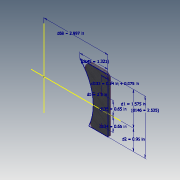
# Autodesk Inventor part: J005357
Saved by Autodesk Inventor 2015 SP1 (Build 190203100, 203)
## iProperties
Created: 2015-07-20
Material: STEEL, LOW CARBON (1008/1018/1020)
Vendor: HHMI: JRC - ID&F
Document SubType Name: Modeling
Designer: ARNOLDJ
Density: 7.85 g/cm^3
Appearance: Metal-Steel (Machined_00)
Mass: 17.3845 g
Surface Area: 65.0391 cm^2
Volume: 14.8586 cm^3
Part Number: J005357
Description: MBS POSITIONER INNER ROTARY LOCK PLATE
Project: P-201804
RuleStatus: InUse
AfterDocSave0: file://Part Number Cleaner
LAB/DEPT: SVOBODA (LAB)
REQUESTING SCIENTIST: SOFRONIEW, NICK
SURFACE ROUGHNESS: 63 Ra
DESIGN DEPARTMENT: HHMI: JRC - ID&F
SPECIAL FINISH: NONE
ALTERED ITEM PART NUMBER: 8131K36
ALTERED ITEM VENDOR: MCMASTER
ALTERED ITEM DESCRIPTION: Nickel-Coated Low-Carbon Steel Rectangular Bar, 1/8" Thick, 2" Width
Author: ARNOLDJ
Revision Number: -
Autodesk Inventor part; units mm, degrees
ref_plane "YZ Plane" through (0, 0, 0) normal (1, 0, 0) x (0, 1, 0)
ref_plane "XZ Plane" through (0, 0, 0) normal (0, 1, 0) x (-1, 0, 0)
ref_plane "XY Plane" through (0, 0, 0) normal (0, 0, 1) x (1, 0, 0)
sketch "Sketch1" plane through (0, 0, 0) normal (0, 0, 1) x (1, 0, 0)
  line L0 (0, 54.7703) -> (0, -37.28) projected
  line L1 (-15.2248, 0) -> (91.3486, 0) projected
  arc A0 (53.2038, -24.13) -> (42.5734, 40.005) centre (0, 0) ccw
  line L2 (42.5734, 40.005) -> (76.1238, 40.005)
  line L3 (76.1238, 40.005) -> (76.1238, -24.13)
  line L4 (53.2038, -24.13) -> (76.1238, -24.13)
  point P0 (68.1228, 16.51)
  point P1 (68.1228, 0)
  point P2 (68.1228, -16.51)
  dimension "d0" = 58.42
  dimension "d1" = 40.005
  dimension "d2" = 24.13
  dimension "d69" = 76.1238
  dimension "d133" = 8.001
  dimension "d134" = 16.51
  dimension "d135" = 16.51
  dimension "d145" = 33.5504
  dimension "d146" = 64.135
  constraints: 6 end point, 2 horizontal, 2 point on circle, 2 vertical alignment, 1 centre point, 1 coincident, 1 perpendicular, 1 point on line
  measures "d0" radius of A0
  measures "d1" distance from line of L2.start L1
  measures "d2" distance from line of L4.start L1
  measures "d69" distance between parallel lines of L0 L3
  measures "d133" distance from line of L3 point (68.123, 16.51)
  measures "d134" distance of point (68.123, -16.51) point (68.123, 0)
  measures "d135" distance of point (68.123, 0) point (68.123, 16.51)
  measures "d145" distance of L2.start L2.end
  measures "d146" distance between parallel lines of L4 L2
extrude "Extrusion1" add sketch "Sketch1" against normal blind 3.175
hole "Hole6" at (68.1228, 16.51, 0) at (68.1228, -16.51, 0) direction (0, 0, -1) diameter 2.4638 end through all
fillet "Fillet11" radius 3.81 1 edges at (53.2038, -24.13, -1.5875)
fillet "Fillet12" radius 6.35 2 edges at (76.1238, 40.005, -1.5875) (42.5734, 40.005, -1.5875)
body "Solid1"
